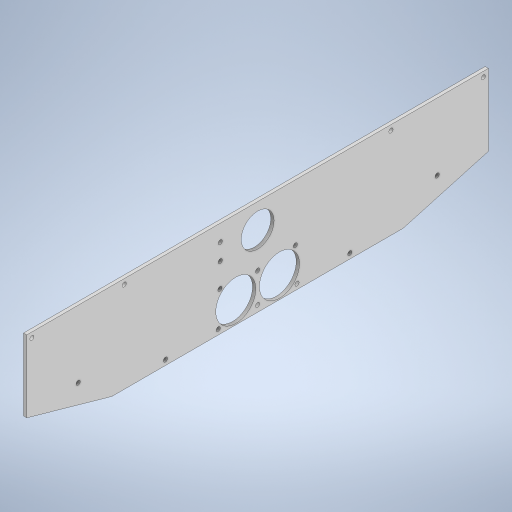
# Autodesk Inventor part: insideChassiPlate2.0
Saved by Autodesk Inventor 2023 (Build 270158000, 158)
## iProperties
Created: 2022-09-08
Part Number: insideChassiPlate2.0
Material: Generic
Document SubType Name: Modeling
Designer: deli
Density: 1 g/cm^3
Appearance: Default
Author: deli
Autodesk Inventor part; units mm, degrees
ref_plane "YZ Plane" through (0, 0, 0) normal (1, 0, 0) x (0, 1, 0)
ref_plane "XZ Plane" through (0, 0, 0) normal (0, 1, 0) x (-1, 0, 0)
ref_plane "XY Plane" through (0, 0, 0) normal (0, 0, 1) x (1, 0, 0)
sketch "Sketch1" plane through (0, 0, 0) normal (1, 0, 0) x (0, 1, 0)
  line L0 (-34.0027, 86.5738) -> (-104.0027, 86.5738) projected
  line L1 (-104.0027, 86.5738) -> (-127.2253, 4.3058) projected
  arc A0 (-127.2253, 4.3058) -> (-127.4133, 2.9475) centre (-122.4133, 2.9475) ccw projected
  line L2 (-127.4133, 2.9475) -> (-127.4133, -279.7999) projected
  arc A1 (-127.4133, -279.7999) -> (-127.2253, -281.1582) centre (-122.4133, -279.7999) ccw projected
  line L3 (-127.2253, -281.1582) -> (-104.0027, -363.4262) projected
  line L4 (-104.0027, -363.4262) -> (-34.0027, -363.4262) projected
  line L5 (-34.0027, -363.4262) -> (-34.0027, -226.9762) projected
  line L6 (-34.0027, -226.9762) -> (230.9973, -226.9762) projected
  line L7 (230.9973, -226.9762) -> (230.9973, -201.5762) projected
  line L8 (230.9973, -201.5762) -> (-34.0027, -201.5762) projected
  line L9 (-34.0027, -201.5762) -> (-34.0027, 86.5738) projected
  circle A2 centre (-66.0027, -101.9662) radius 2 projected
  circle A3 centre (-122.4133, -228.31) radius 2 projected
  circle A4 centre (-122.4133, -48.5424) radius 2 projected
  circle A5 centre (-39.0027, -8.4262) radius 2 projected
  circle A6 centre (-39.0027, -358.4262) radius 2 projected
  circle A7 centre (-89.2685, -175.1441) radius 2 projected
  circle A8 centre (-99.4133, 36.5738) radius 2 projected
  circle A9 centre (-99.4133, -313.4262) radius 2 projected
  circle A10 centre (-106.6633, -117.135) radius 7 projected
  circle A11 centre (-106.6633, -159.7175) radius 7 projected
  circle A12 centre (-92.1807, -138.4262) radius 2 projected
  circle A13 centre (-121.1459, -138.4262) radius 2 projected
  circle A14 centre (-122.4133, -100.0323) radius 2 projected
  circle A15 centre (-122.4133, -176.8201) radius 2 projected
  circle A16 centre (-39.0027, 81.5738) radius 2 projected
  circle A17 centre (-89.2685, -101.7083) radius 2 projected
  circle A18 centre (-39.0027, -268.4262) radius 2 projected
  circle A19 centre (222.9973, -212.6887) radius 2 projected
  circle A20 centre (-58.0027, -138.4262) radius 16 projected
  circle A21 centre (-50.0027, -101.9662) radius 2 projected
  line L10 (-34.0027, -201.5762) -> (-34.0027, -226.9762)
  circle A22 centre (-106.6633, -117.135) radius 19.5
  circle A23 centre (-106.6633, -159.7175) radius 19.5
  dimension "d6" = 39
  dimension "d7" = 39
  constraints: 2 centre point, 2 coincident, 2 end point, 1 vertical
  measures "d6" diameter of A22
  measures "d7" diameter of A23
extrude "Extrusion1" add sketch "Sketch1" along normal blind 3.175 contours L9 L10 L5 L4 L3 A1 L2 A0 L1 L0
body "Solid1"
